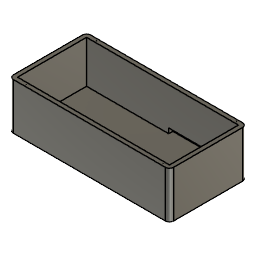
Encapsulado proyecto (Autodesk Fusion 360 design; units mm, degrees)
part number: 2026-06-22-13-33-49-175
Autodesk Fusion 360 part; units mm, degrees
sketch "Boceto1" plane through (0, 0, 0) normal (0, 0, 1) x (1, 0, 0)
  line L0 (96.4, 46.5) -> (-96.4, 46.5)
  line L1 (-96.4, 46.5) -> (-96.4, -46.5)
  line L2 (-96.4, -46.5) -> (96.4, -46.5)
  line L3 (96.4, -46.5) -> (96.4, 46.5)
  line L4 (96.4, 46.5) -> (-96.4, -46.5) construction
  line L5 (-96.4, 46.5) -> (96.4, -46.5) construction
  dimension "d1" = 192.8
  dimension "d2" = 93
  constraint horizontal L0
  constraint perpendicular L0 L1
  constraint parallel L0 L2
  constraint parallel L1 L3
  constraint coincident L4 origin
  constraint coincident L5 origin
  measures "d1" distance of L1.end L2.end
  measures "d2" distance of L0.end L1.end
extrude "Extruir1" add sketch "Boceto1" along normal blind 56
shell "Vaciado1" thickness 5 removed faces 1 at (-32.1333, 15.5, 56)
fillet "Empalme1" radius 5 1 edges at (96.4, 46.5, 28)
fillet "Empalme2" radius 5 1 edges at (96.4, -46.5, 28)
fillet "Empalme3" radius 5 1 edges at (-96.4, -46.5, 28)
fillet "Empalme4" radius 5 1 edges at (-96.4, 46.5, 28)
sketch "Boceto3" plane through (0, 46.5, 0) normal (0, 1, 0) x (-1, 0, 0)
  line L0 (91.4, 0) -> (91.4, 56)
  line L1 (91.4, 56) -> (-91.4, 56)
  line L2 (-91.4, 56) -> (-91.4, 0)
  line L3 (-91.4, 0) -> (91.4, 0)
  line L4 (-91.4, 0) -> (-91.4, 5)
  line L5 (-91.4, 5) -> (-48.4, 5)
  line L6 (-48.4, 5) -> (-7.4, 5)
  line L7 (-7.4, 5) -> (-7.4, 11)
  line L8 (-7.4, 11) -> (-48.4, 11)
  line L9 (-48.4, 11) -> (-48.4, 5)
  dimension "d17" = 5
  dimension "d18" = 43
  dimension "d19" = 41
  dimension "d20" = 6
  dimension "d21" = 41
  constraint coincident L2.end L3.start
  constraint perpendicular L3 L4
  constraint perpendicular L2 L5
  constraint perpendicular L2 L6
  constraint perpendicular L3 L7
  constraint perpendicular L2 L8
  measures "d17" distance of L2.end L4.end
  measures "d18" distance of L4.end L5.end
  measures "d19" distance of L5.end L6.end
  measures "d20" distance of L6.end L7.end
  measures "d21" distance of L7.end L8.end
extrude "Extruir2" cut sketch "Boceto3" against normal blind 5 contours L6 L7 L8 L9
sketch "Boceto4" plane through (0, 0, 56) normal (0, 0, 1) x (-1, 0, 0)
  arc A0 (91.4, -46.5) -> (96.4, -41.5) centre (91.4, -41.5) ccw
  line L0 (96.4, -41.5) -> (96.4, 41.5)
  arc A1 (96.4, 41.5) -> (91.4, 46.5) centre (91.4, 41.5) ccw
  line L1 (91.4, 46.5) -> (-91.4, 46.5)
  arc A2 (-91.4, 46.5) -> (-96.4, 41.5) centre (-91.4, 41.5) ccw
  line L2 (-96.4, 41.5) -> (-96.4, -41.5)
  arc A3 (-96.4, -41.5) -> (-91.4, -46.5) centre (-91.4, -41.5) ccw
  line L3 (-91.4, -46.5) -> (91.4, -46.5)
  line L4 (-91.4, 41.5) -> (91.4, 41.5)
  line L5 (91.4, 41.5) -> (91.4, -41.5)
  line L6 (91.4, -41.5) -> (-91.4, -41.5)
  line L7 (-91.4, -41.5) -> (-91.4, 41.5)
  line L8 (-96.4, -46.5) -> (-86.4, -46.5)
  line L9 (-86.4, -46.5) -> (-86.4, -44)
  dimension "d24" = 10
  dimension "d25" = 2.5
  constraint parallel L3 L8
  constraint perpendicular L6 L9
  measures "d24" distance of L8.start L8.end
  measures "d25" distance of L8.end L9.end
sketch "Boceto5" plane through (0, 0, 0) normal (0, 0, 1) x (1, 0, 0)
sketch "Boceto6" plane through (0, 0, 56) normal (0, 0, 1) x (-1, 0, 0)
sketch "Boceto7" plane through (0, 0, 56) normal (0, 0, 1) x (-1, 0, 0)
hole "Agujero1" at (86.4, 44, 56) direction (0, 0, -1) diameter 0.769 depth 2 tip angle 118
thread "Rosca1" "ISO Metric profile 1.0 M1x0.25 M1x0.25 6H" thread offset 0 thread depth 7.4
sketch "Boceto8" plane through (0, 0, 0) normal (0, 0, 1) x (1, 0, 0)
sketch "Boceto9" plane through (0, 0, 56) normal (0, 0, 1) x (-1, 0, 0)
  circle A0 centre (-86.4, -44) radius 0.3847
  arc A1 (91.4, -46.5) -> (96.4, -41.5) centre (91.4, -41.5) ccw
  line L0 (96.4, -41.5) -> (96.4, 41.5)
  arc A2 (96.4, 41.5) -> (91.4, 46.5) centre (91.4, 41.5) ccw
  line L1 (91.4, 46.5) -> (-91.4, 46.5)
  arc A3 (-91.4, 46.5) -> (-96.4, 41.5) centre (-91.4, 41.5) ccw
  line L2 (-96.4, 41.5) -> (-96.4, -41.5)
  arc A4 (-96.4, -41.5) -> (-91.4, -46.5) centre (-91.4, -41.5) ccw
  line L3 (-91.4, -46.5) -> (91.4, -46.5)
  line L4 (-91.4, 41.5) -> (91.4, 41.5)
  line L5 (91.4, 41.5) -> (91.4, -41.5)
  line L6 (91.4, -41.5) -> (-91.4, -41.5)
  line L7 (-91.4, -41.5) -> (-91.4, 41.5)
  line L8 (81.8102, -46.5) -> (81.8102, -44)
  dimension "d31" = 2.5
  constraint coincident L3 L8.start
  constraint perpendicular L6 L8
  measures "d31" distance of L8.start L8.end
hole "Agujero2" at (-81.8102, 44, 56) direction (0, 0, -1) diameter 0.769 depth 2 tip angle 118
thread "Rosca2" "ISO Metric profile 1.0 M1x0.25 M1x0.25 6H" thread offset 0 thread depth 7.4
sketch "Boceto10" plane through (0, 0, 56) normal (0, 0, 1) x (-1, 0, 0)
  circle A0 centre (81.8102, -44) radius 0.3847
  circle A1 centre (-86.4, -44) radius 0.3847
  arc A2 (91.4, -46.5) -> (96.4, -41.5) centre (91.4, -41.5) ccw
  line L0 (96.4, -41.5) -> (96.4, 41.5)
  arc A3 (96.4, 41.5) -> (91.4, 46.5) centre (91.4, 41.5) ccw
  line L1 (91.4, 46.5) -> (-91.4, 46.5)
  arc A4 (-91.4, 46.5) -> (-96.4, 41.5) centre (-91.4, 41.5) ccw
  line L2 (-96.4, 41.5) -> (-96.4, -41.5)
  arc A5 (-96.4, -41.5) -> (-91.4, -46.5) centre (-91.4, -41.5) ccw
  line L3 (-91.4, -46.5) -> (91.4, -46.5)
  line L4 (-91.4, 41.5) -> (91.4, 41.5)
  line L5 (91.4, 41.5) -> (91.4, -41.5)
  line L6 (91.4, -41.5) -> (-91.4, -41.5)
  line L7 (-91.4, -41.5) -> (-91.4, 41.5)
  line L8 (78.4029, 46.5) -> (78.4029, 44)
  line L9 (-85.7578, 46.5) -> (-85.7578, 44)
  dimension "d37" = 2.5
  dimension "d38" = 2.5
  constraint coincident L1 L8.start
  constraint perpendicular L4 L8
  constraint coincident L1 L9.start
  constraint perpendicular L4 L9
  measures "d37" distance of L8.start L8.end
  measures "d38" distance of L9.start L9.end
hole "Agujero3" at (-78.4029, -44, 56) direction (0, 0, -1) diameter 0.769 depth 2 tip angle 118
thread "Rosca3" "ISO Metric profile 1.0 M1x0.25 M1x0.25 6H" thread offset 0 thread depth 7.4
sketch "Boceto11" plane through (0, 0, 56) normal (0, 0, 1) x (-1, 0, 0)
  circle A0 centre (78.4029, 44) radius 0.3847
  circle A1 centre (81.8102, -44) radius 0.3847
  circle A2 centre (-86.4, -44) radius 0.3847
  arc A3 (91.4, -46.5) -> (96.4, -41.5) centre (91.4, -41.5) ccw
  line L0 (96.4, -41.5) -> (96.4, 41.5)
  arc A4 (96.4, 41.5) -> (91.4, 46.5) centre (91.4, 41.5) ccw
  line L1 (91.4, 46.5) -> (-91.4, 46.5)
  arc A5 (-91.4, 46.5) -> (-96.4, 41.5) centre (-91.4, 41.5) ccw
  line L2 (-96.4, 41.5) -> (-96.4, -41.5)
  arc A6 (-96.4, -41.5) -> (-91.4, -46.5) centre (-91.4, -41.5) ccw
  line L3 (-91.4, -46.5) -> (91.4, -46.5)
  line L4 (-91.4, 41.5) -> (91.4, 41.5)
  line L5 (91.4, 41.5) -> (91.4, -41.5)
  line L6 (91.4, -41.5) -> (-91.4, -41.5)
  line L7 (-91.4, -41.5) -> (-91.4, 41.5)
  line L8 (-86.4, 46.5) -> (-86.4, 44)
  dimension "d44" = 2.5
  constraint coincident L1 L8.start
  constraint perpendicular L4 L8
  measures "d44" distance of L8.start L8.end
hole "Agujero4" at (86.4, -44, 56) direction (0, 0, -1) diameter 0.769 depth 2 tip angle 118
thread "Rosca4" "ISO Metric profile 1.0 M1x0.25 M1x0.25 6H" thread offset 0 thread depth 7.4
